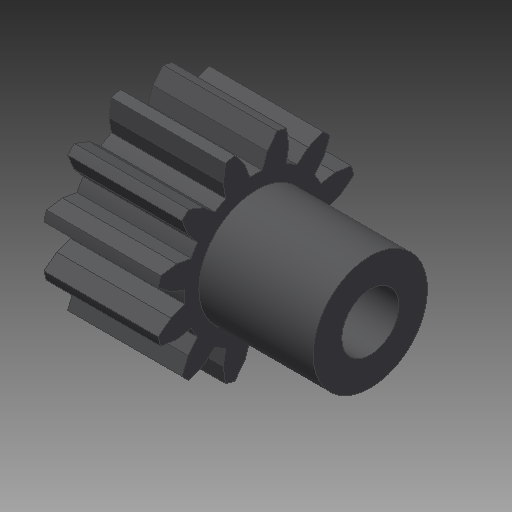
# Autodesk Inventor part: M-0.5 Zb-4mm M-0.7 Zb-5mm mN 21101200
Saved by Autodesk Inventor 2017.3 (Build 213256000, 256)
## iProperties
Category: PARTsolutions
Company: MAEDLER
Created: 2018-07-09
Part Number: M-0.5 Zb-4mm M-0.7 Zb-5mm mN 21101200
Catalog Web Link: www.cadenas.de
Description: M-0.5 Zb-4mm M-0.7 Zb-5mm mN-Spur Gears, Steel, Module 0.5 and 0,7
Vendor: MAEDLER
Document SubType Name: Modeling
Designer: psAdmin
Manufacturer: MAEDLER
Mass: 1 g
Surface Area: 2.90871 cm^2
Volume: 0.136832 cm^3
Density: 1 g/cm^3
Material: Allgemein
Appearance: PSOLRGB-175-175-175
PSOL_IDENT_0: {$CADENAS_DATA\23d-libs\maedler\antriebselemente\stirnzahnraeder\stirnzahnraeder_stahl\modul_0.5_und
PSOL_IDENT_1: _0.7\m-0.5_zb-4mm_m-0.7_zb-5mm_mn.prj},238 {VTYP=3D},{NB=M-0.5 Zb-4mm M-0.7 Zb-5mm mN 21101200},{LIN
PSOL_IDENT_2: A=M-0.5 Zb-4mm M-0.7 Zb-5mm mN 21101200},{NN=M-0.5 Zb-4mm M-0.7 Zb-5mm mN},{DATE=27.10.2015 07:21:56
PSOL_IDENT_3: },{GEOMDATE=11.05.2009 09:51:00},{VERSION=},{LINEID=20},{LINESUBID=-1},{WBVAR=}  {NB=M-0.5 Zb-4mm M-
PSOL_IDENT_4: 0.7 Zb-5mm mN 21101200},{LINA=M-0.5 Zb-4mm M-0.7 Zb-5mm mN 21101200},{KT=DUMMY},{ARTNR=21101200},{WS
PSOL_IDENT_5: T=11SMnPb30},{M=0.5},{Z=12},{PDF=PDF Katalogseite},{B1=4.0},{DA=7.00},{D=6.00},{NL=4},{ND=4},{B=2},{
PSOL_IDENT_6: MD=1.0},{GEW=1.000}
NN: M-0.5 Zb-4mm M-0.7 Zb-5mm mN
NT: Spur Gears, Steel, Module 0.5 and 0,7
NB: M-0.5 Zb-4mm M-0.7 Zb-5mm mN 21101200
NBSYN: M-0.5 Zb-4mm M-0.7 Zb-5mm mN $ARTNR.
LINA: M-0.5 Zb-4mm M-0.7 Zb-5mm mN 21101200
ARTNR: 21101200
WST: 11SMnPb30
M: 0.5
Z: 12
PDF: PDF Katalogseite
B1: 4.0
DA: 7.00
D: 6.00
NL: 4
ND: 4
B: 2
MD: 1.0
GEW: 1.000
SUPPLIER: MAEDLER
ARTICLENO: M-0.5 Zb-4mm M-0.7 Zb-5mm mN 21101200
BOMINFO: M-0.5 Zb-4mm M-0.7 Zb-5mm mN 21101200
CREATOR: CADENAS GmbH
Title: M-0.5 Zb-4mm M-0.7 Zb-5mm mN 21101200
Author: Cadenas PARTsolutions
Comments: Spur Gears, Steel, Module 0.5 and 0,7
Autodesk Inventor part; units mm, degrees
ref_plane "YZ Plane" through (0, 0, 0) normal (1, 0, 0) x (0, 1, 0)
ref_plane "XZ Plane" through (0, 0, 0) normal (0, 1, 0) x (-1, 0, 0)
ref_plane "XY Plane" through (0, 0, 0) normal (0, 0, 1) x (1, 0, 0)
sketch "Skizze_1" plane through (0, 0, 0) normal (1, 0, 0) x (0, 1, 0)
  arc A0 (-0.7439, 3.42) -> (-1.0658, 3.3338) centre (0, 0) ccw
  line L0 (-1.0658, 3.3338) -> (-1.1459, 2.7725)
  line L1 (-1.1459, 2.7725) -> (-1.0565, 2.2658)
  arc A1 (-1.0565, 2.2658) -> (-1.4339, 2.0479) centre (0, 0) ccw
  line L2 (-1.4339, 2.0479) -> (-1.8281, 2.3786)
  line L3 (-1.8281, 2.3786) -> (-2.3542, 2.5899)
  arc A2 (-2.3542, 2.5899) -> (-2.5899, 2.3542) centre (0, 0) ccw
  line L4 (-2.5899, 2.3542) -> (-2.3786, 1.8281)
  line L5 (-2.3786, 1.8281) -> (-2.0479, 1.4339)
  arc A3 (-2.0479, 1.4339) -> (-2.2658, 1.0565) centre (0, 0) ccw
  line L6 (-2.2658, 1.0565) -> (-2.7725, 1.1459)
  line L7 (-2.7725, 1.1459) -> (-3.3338, 1.0658)
  arc A4 (-3.3338, 1.0658) -> (-3.42, 0.7439) centre (0, 0) ccw
  line L8 (-3.42, 0.7439) -> (-2.974, 0.3939)
  line L9 (-2.974, 0.3939) -> (-2.4905, 0.2179)
  arc A5 (-2.4905, 0.2179) -> (-2.4905, -0.2179) centre (0, 0) ccw
  line L10 (-2.4905, -0.2179) -> (-2.974, -0.3939)
  line L11 (-2.974, -0.3939) -> (-3.42, -0.7439)
  arc A6 (-3.42, -0.7439) -> (-3.3338, -1.0658) centre (0, 0) ccw
  line L12 (-3.3338, -1.0658) -> (-2.7725, -1.1459)
  line L13 (-2.7725, -1.1459) -> (-2.2658, -1.0565)
  arc A7 (-2.2658, -1.0565) -> (-2.0479, -1.4339) centre (0, 0) ccw
  line L14 (-2.0479, -1.4339) -> (-2.3786, -1.8281)
  line L15 (-2.3786, -1.8281) -> (-2.5899, -2.3542)
  arc A8 (-2.5899, -2.3542) -> (-2.3542, -2.5899) centre (0, 0) ccw
  line L16 (-2.3542, -2.5899) -> (-1.8281, -2.3786)
  line L17 (-1.8281, -2.3786) -> (-1.4339, -2.0479)
  arc A9 (-1.4339, -2.0479) -> (-1.0565, -2.2658) centre (0, 0) ccw
  line L18 (-1.0565, -2.2658) -> (-1.1459, -2.7725)
  line L19 (-1.1459, -2.7725) -> (-1.0658, -3.3338)
  arc A10 (-1.0658, -3.3338) -> (-0.7439, -3.42) centre (0, 0) ccw
  line L20 (-0.7439, -3.42) -> (-0.3939, -2.974)
  line L21 (-0.3939, -2.974) -> (-0.2179, -2.4905)
  arc A11 (-0.2179, -2.4905) -> (0.2179, -2.4905) centre (0, 0) ccw
  line L22 (0.2179, -2.4905) -> (0.3939, -2.974)
  line L23 (0.3939, -2.974) -> (0.7439, -3.42)
  arc A12 (0.7439, -3.42) -> (1.0658, -3.3338) centre (0, 0) ccw
  line L24 (1.0658, -3.3338) -> (1.1459, -2.7725)
  line L25 (1.1459, -2.7725) -> (1.0565, -2.2658)
  arc A13 (1.0565, -2.2658) -> (1.4339, -2.0479) centre (0, 0) ccw
  line L26 (1.4339, -2.0479) -> (1.8281, -2.3786)
  line L27 (1.8281, -2.3786) -> (2.3542, -2.5899)
  arc A14 (2.3542, -2.5899) -> (2.5899, -2.3542) centre (0, 0) ccw
  line L28 (2.5899, -2.3542) -> (2.3786, -1.8281)
  line L29 (2.3786, -1.8281) -> (2.0479, -1.4339)
  arc A15 (2.0479, -1.4339) -> (2.2658, -1.0565) centre (0, 0) ccw
  line L30 (2.2658, -1.0565) -> (2.7725, -1.1459)
  line L31 (2.7725, -1.1459) -> (3.3338, -1.0658)
  arc A16 (3.3338, -1.0658) -> (3.42, -0.7439) centre (0, 0) ccw
  line L32 (3.42, -0.7439) -> (2.974, -0.3939)
  line L33 (2.974, -0.3939) -> (2.4905, -0.2179)
  arc A17 (2.4905, -0.2179) -> (2.4905, 0.2179) centre (0, 0) ccw
  line L34 (2.4905, 0.2179) -> (2.974, 0.3939)
  line L35 (2.974, 0.3939) -> (3.42, 0.7439)
  arc A18 (3.42, 0.7439) -> (3.3338, 1.0658) centre (0, 0) ccw
  line L36 (3.3338, 1.0658) -> (2.7725, 1.1459)
  line L37 (2.7725, 1.1459) -> (2.2658, 1.0565)
  arc A19 (2.2658, 1.0565) -> (2.0479, 1.4339) centre (0, 0) ccw
  line L38 (2.0479, 1.4339) -> (2.3786, 1.8281)
  line L39 (2.3786, 1.8281) -> (2.5899, 2.3542)
  arc A20 (2.5899, 2.3542) -> (2.3542, 2.5899) centre (0, 0) ccw
  line L40 (2.3542, 2.5899) -> (1.8281, 2.3786)
  line L41 (1.8281, 2.3786) -> (1.4339, 2.0479)
  arc A21 (1.4339, 2.0479) -> (1.0565, 2.2658) centre (0, 0) ccw
  line L42 (1.0565, 2.2658) -> (1.1459, 2.7725)
  line L43 (1.1459, 2.7725) -> (1.0658, 3.3338)
  arc A22 (1.0658, 3.3338) -> (0.7439, 3.42) centre (0, 0) ccw
  line L44 (0.7439, 3.42) -> (0.3939, 2.974)
  line L45 (0.3939, 2.974) -> (0.2179, 2.4905)
  arc A23 (0.2179, 2.4905) -> (-0.2179, 2.4905) centre (0, 0) ccw
  line L46 (-0.2179, 2.4905) -> (-0.3939, 2.974)
  line L47 (-0.3939, 2.974) -> (-0.7439, 3.42)
  constraints: 96 end point, 48 point on circle, 24 centre point
extrude "Extrusion1" add sketch "Skizze_1" along normal mid plane 4
sketch "Skizze_2" plane through (0, 0, 0) normal (0, 0, 1) x (1, 0, 0)
  line L0 (6, 0) -> (2, 0)
  line L1 (2, 0) -> (2, 2)
  line L2 (2, 2) -> (6, 2)
  line L3 (6, 2) -> (6, 0)
  line L4 (6, 0) -> (2, 0)
  constraints: 10 end point
revolve "Revolution1" add sketch "Skizze_2" angle 360 about axis through (6, 0, 0) along (1, 0, 0)
sketch "Skizze_3" plane through (6, 0, 0) normal (1, 0, 0) x (0, 1, 0)
  circle A0 centre (0, 0) radius 1
  constraints: 1 centre point
extrude "Extrusion2" cut sketch "Skizze_3" along normal mid plane 16
body "Solid1"
